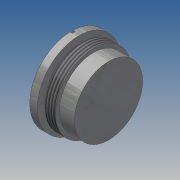
# Autodesk Inventor part: Gehäusedeckel_ra8846s
Saved by Autodesk Inventor 2021 (Build 250183000, 183)
## iProperties
Created: 2020-11-17
Part Number: Gehäusedeckel_ra8846s
Material: Stahl, unlegiert
Document SubType Name: Modeling
Designer: Ricardo A
Density: 7.85 g/cm^3
Appearance: Stahl
Description: Motor_Teil10_Gehäused
Mass: 10.0417 g
Surface Area: 19.1309 cm^2
Volume: 1.2792 cm^3
Author: Sander
Revision Number: Rev00
Autodesk Inventor part; units mm, degrees
ref_plane "YZ-Ebene" through (0, 0, 0) normal (1, 0, 0) x (0, 1, 0)
ref_plane "XZ-Ebene" through (0, 0, 0) normal (0, 1, 0) x (-1, 0, 0)
ref_plane "XY-Ebene" through (0, 0, 0) normal (0, 0, 1) x (1, 0, 0)
sketch "Skizze1" plane through (0, 0, 0) normal (0, 0, 1) x (1, 0, 0)
  line L0 (-1.96, 0) -> (11.76, 0) projected
  line L1 (0, -2.2) -> (0, 13.2) projected
  line L2 (8, 0) -> (8, 8)
  line L3 (8, 8) -> (0, 8)
  line L4 (9.8, 0) -> (9.8, 9)
  line L5 (9.8, 9) -> (5.8, 9)
  line L6 (0, 11) -> (2, 11)
  line L7 (5.8, 9) -> (5.8, 10)
  line L8 (2, 11) -> (2, 9)
  line L9 (5.8, 10) -> (3, 10)
  line L10 (3, 10) -> (3, 9)
  arc A0 (2, 9) -> (3, 9) centre (2.5, 9) ccw
  point P0 (0, 0)
  dimension "d8" = 9
  dimension "d9" = 9.8
  dimension "d10" = 8
  dimension "d12" = 8
  dimension "d13" = 4
  dimension "d14" = 2
  dimension "d15" = 11
  dimension "d17" = 0.5
  dimension "d18" = 9
  dimension "d19" = 10
  constraints: 18 end point, 4 vertical, 3 horizontal, 3 point on line, 2 perpendicular, 2 point on circle, 2 tangent, 1 centre point, 1 horizontal alignment
  measures "d8" distance of L4.start L4.end
  measures "d9" distance of L4.start point (0, 0)
  measures "d10" distance from line of L2 point (0, 0)
  measures "d12" distance of L2.start L2.end
  measures "d13" distance of L4.end L5.end
  measures "d14" distance of L6.start L6.end
  measures "d15" distance from line of point (0, 0) L6
  measures "d17" radius of A0
  measures "d18" vertical distance of point (0, 0) A0.centre
  measures "d19" distance from line of L0 L7.end
revolve "Umdrehung1" add sketch "Skizze1" angle 360 about axis through (-10, 0, 0) along (1, 0, 0) contours L2 L3 L1 L6 L8 A0 L10 L9 L7 L5 L4 L0
sketch "Skizze2" plane through (0, 0, 0) normal (-1, 0, 0) x (0, 0, 1)
  circle A0 centre (0, 0) radius 8 projected
  circle A1 centre (0, 0) radius 11 projected
  circle A2 centre (0, 0) radius 8 projected
  line L0 (-15.4, 0) -> (15.4, 0) projected
  line L1 (10.9927, 0.4) -> (-10.9927, 0.4)
  line L2 (10.9927, -0.4) -> (-10.9927, -0.4)
  point P0 (-7.99, 0.4)
  point P1 (-7.99, -0.4)
  point P2 (7.99, 0.4)
  point P3 (7.99, -0.4)
  dimension "d23" = 0.8
  constraints: 4 end point, 4 point on circle, 1 horizontal, 1 parallel, 1 other
  measures "d23" distance between parallel lines of L2 L1
extrude "Extrusion1" cut sketch "Skizze2" against normal blind 0.6 contours L0 A1 L2 A0 | A0 L1 A1 L0 | L0 A1 L1 A0 | A0 L2 A1 L0
thread "Gewinde1" size "M20x0.75" class "6g" standard "ISO Metric profile" full length
